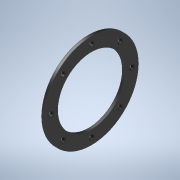
# Autodesk Inventor part: MountingRing
Saved by Autodesk Inventor 2020 (Build 240168000, 168)
## iProperties
Created: 2019-11-13
Part Number: MountingRing
Material: Generic
Document SubType Name: Modeling
Designer: nicoc
Density: 1 g/cm^3
Appearance: Glossy - Black
Author: nicoc
Autodesk Inventor part; units mm, degrees
ref_plane "YZ Plane" through (0, 0, 0) normal (1, 0, 0) x (0, 1, 0)
ref_plane "XZ Plane" through (0, 0, 0) normal (0, 1, 0) x (-1, 0, 0)
ref_plane "XY Plane" through (0, 0, 0) normal (0, 0, 1) x (1, 0, 0)
sketch "Sketch1" plane through (0, 0, 0) normal (1, 0, 0) x (0, 1, 0)
  circle A0 centre (175, -175) radius 175
  point P0 (0, 0)
  dimension "d0" = 175
  dimension "d1" = 175
  dimension "d2" = 350
  constraints: 1 centre point
  measures "d0" horizontal distance of A0.centre point (0, 0)
  measures "d1" horizontal distance of A0.centre point (0, 0)
  measures "d2" diameter of A0
extrude "Extrusion1" add sketch "Sketch1" along normal blind 10
sketch "Sketch2" plane through (10, 175, -175) normal (1, 0, 0) x (0, 0, -1)
  circle A0 centre (0, 0) radius 125
  point P0 (-175, -175)
  dimension "d5" = 250
  constraints: 1 centre point
  measures "d5" diameter of A0
extrude "Extrusion2" cut sketch "Sketch2" against normal through all
sketch "Sketch3" plane through (10, 175, -175) normal (1, 0, 0) x (0, 0, -1)
  circle A0 centre (0, 0) radius 175 projected
  point P0 (-175, -175)
  point P1 (-150, 0)
  dimension "d8" = 150
  dimension "d9" = 0
  measures "d8" distance of A0.centre point (-150, 0)
  measures "d9" vertical distance of A0.centre point (-150, 0)
hole "Hole1" at (10, 175, -25) direction (-1, 0, 0) diameter 17 end through all
pattern_circular "Circular Pattern1" count 8 over 360 about axis through (10, 175, -175) along (-1, 0, 0) of "Hole1"
body "Solid1"
